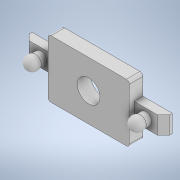
# Autodesk Inventor part: motor_cover
Saved by Autodesk Inventor 2022.1 (Build 261234000, 234)
## iProperties
Created: 2021-07-13
Part Number: motor_cover
Material: Generic
Document SubType Name: Modeling
Designer: dwbertol
Density: 1 g/cm^3
Appearance: Default
Author: dwbertol
## iProperties of the stored document motor_cover_3DPrint.ipt
Created: 2021-07-17
Part Number: motor_cover_3DPrint
Material: Generic
Document SubType Name: Modeling
Designer: dwbertol
Density: 1 g/cm^3
Appearance: Default
Author: dwbertol
Autodesk Inventor part; units mm, degrees
ref_plane "YZ Plane" through (0, 0, 0) normal (1, 0, 0) x (0, 1, 0)
ref_plane "XZ Plane" through (0, 0, 0) normal (0, 1, 0) x (-1, 0, 0)
ref_plane "XY Plane" through (0, 0, 0) normal (0, 0, 1) x (1, 0, 0)
sketch "Sketch1" plane through (0, 0, 0) normal (0, 0, 1) x (1, 0, 0)
  line L0 (-6.9, 4.9) -> (6.9, 4.9)
  line L1 (6.9, 4.9) -> (6.9, -4.9)
  line L2 (6.9, -4.9) -> (-6.9, -4.9)
  line L3 (-6.9, -4.9) -> (-6.9, 4.9)
  circle A0 centre (0, 0) radius 1.925
  line L4 (-6.9, -1.5) -> (-11.9, -1.5)
  line L5 (-11.9, -1.5) -> (-11.9, 1.5)
  line L6 (-11.9, 1.5) -> (-6.9, 1.5)
  line L7 (-6.9, 1.5) -> (-6.9, -1.5)
  line L8 (6.9, -1.5) -> (11.9, -1.5)
  line L9 (11.9, -1.5) -> (11.9, 1.5)
  line L10 (11.9, 1.5) -> (6.9, 1.5)
  line L11 (6.9, 1.5) -> (6.9, -1.5)
  dimension "d0" = 13.8
  dimension "d1" = 9.8
  dimension "d2" = 6.9
  dimension "d3" = 4.9
  dimension "d6" = 3.85
  dimension "d7" = 3
  dimension "d8" = 1.5
  dimension "d9" = 5
  dimension "d10" = 5
  constraints: 24 end point, 6 parallel, 3 horizontal, 3 perpendicular, 2 collinear, 2 point on line, 1 centre point, 1 coincident
  measures "d0" distance between parallel lines of L1 L3
  measures "d1" distance between parallel lines of L0 L2
  measures "d2" distance from line of L3 point (0, 0)
  measures "d3" distance from line of point (0, 0) L0
  measures "d6" diameter of A0
  measures "d7" distance between parallel lines of L4 L6
  measures "d8" distance from line of point (0, 0) L4
  measures "d9" distance between parallel lines of L3 L5
  measures "d10" distance between parallel lines of L11 L9
extrude "Extrusion1" add sketch "Sketch1" along normal blind 2.3 contours L0 L1 L2 L3
extrude "Extrusion2" add sketch "Sketch1" along normal blind 1.5 contours L3 L4 L5 L6 | L10 L9 L8 L1
chamfer "Chamfer1" distance 1 angle 45 2 edges at (-11.9, 0, 1.5) (11.9, 0, 1.5)
sketch "Sketch2" plane through (0, 0, 1.5) normal (0, 0, 1) x (1, 0, 0)
  circle A0 centre (8.9, 0) radius 1
  line L0 (10.9, 1.5) -> (6.9, 1.5) projected
  line L1 (0, 0) -> (0.8425, 0) construction
  line L2 (6.9, -4.9) -> (6.9, 4.9) projected
  circle A1 centre (-8.9, 0) radius 1
  line L3 (-6.9, 4.9) -> (-6.9, -4.9) projected
  dimension "d17" = 2
  dimension "d19" = 2
  dimension "d20" = 2
  dimension "d21" = 2
  constraints: 2 centre point, 2 end point, 2 point on line, 1 horizontal
  measures "d17" diameter of A0
  measures "d19" distance from line of L2 A0.centre
  measures "d20" diameter of A1
  measures "d21" distance from line of L3 A1.centre
extrude "Extrusion3" add sketch "Sketch2" along normal blind 1.5
sketch "Sketch3" plane through (0, 0, 0) normal (0, 1, 0) x (-1, 0, 0)
  line L0 (9.9, 3) -> (7.9, 3) projected
  circle A0 centre (8.9, 3) radius 1.15
  line L1 (7.9, 1.5) -> (7.9, 3) projected
  line L2 (9.9, 1.5) -> (9.9, 3) projected
  line L3 (-7.9, 3) -> (-9.9, 3) projected
  circle A1 centre (-8.9, 3) radius 1.15
  line L4 (-9.9, 1.5) -> (-9.9, 3) projected
  line L5 (9.9, 3) -> (10.05, 3)
  line L6 (7.9, 3) -> (7.75, 3)
  line L7 (-7.75, 3) -> (-10.05, 3)
  point P0 (0, 0)
  dimension "d24" = 0.15
  dimension "d25" = 0.15
  constraints: 6 end point, 4 point on circle, 2 centre point, 2 collinear, 2 midpoint, 1 horizontal, 1 point on line
  measures "d24" distance edge to line of A0 L1
  measures "d25" distance edge to line of A1 L4
revolve "Revolution1" add sketch "Sketch3" angle 360 about axis through (-9.9, 0, 3) along (-1, 0, 0) contours L0 L6 A0 L5 | L3 L7 A1
fillet "Fillet1" radius 0.5 4 edges at (-6.9, -4.9, 1.15) (-6.9, 4.9, 1.15) (6.9, 4.9, 1.15) (6.9, -4.9, 1.15)
equation "\"d2\" = 0.5 * d0"
equation "\"d3\" = 0.5 * d1"
equation "\"d8\" = 0.5 * d7"
equation "\"d10\" = d9"
equation "\"d20\" = d17"
equation "\"d21\" = d19"
body "Solid1"
